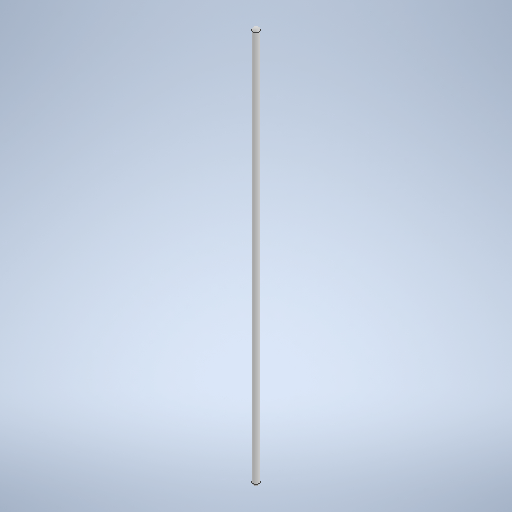
# Autodesk Inventor part: 8 mm rod (50 cm)
Saved by Autodesk Inventor 2025 (Build 290162000, 162)
## iProperties
Created: 2024-06-26
Part Number: 8 mm rod (50 cm)
Material: Generic
Document SubType Name: Modeling
Designer: User
Density: 1 g/cm^3
Appearance: Default
Author: User
Autodesk Inventor part; units mm, degrees
ref_plane "YZ Plane" through (0, 0, 0) normal (1, 0, 0) x (0, 1, 0)
ref_plane "XZ Plane" through (0, 0, 0) normal (0, 1, 0) x (-1, 0, 0)
ref_plane "XY Plane" through (0, 0, 0) normal (0, 0, 1) x (1, 0, 0)
sketch "Sketch1" plane through (0, 0, 0) normal (0, 1, 0) x (-1, 0, 0)
  circle A0 centre (0, 0) radius 4
  dimension "d1" = 8
  constraints: 1 centre point, 1 coincident
  measures "d1" diameter of A0
extrude "Extrusion1" add sketch "Sketch1" along normal mid plane 500
fillet "Fillet1" radius 4 2 edges at (4, 250, 0) (4, -250, 0)
body "Solid1"
